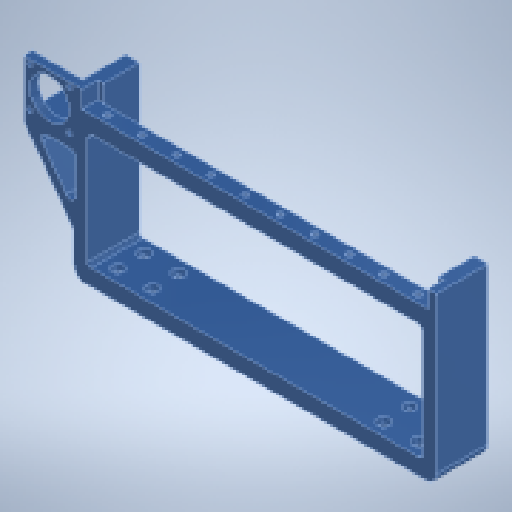
# Autodesk Inventor part: gantry_R
Saved by Autodesk Inventor 2024.1 (Build 281209000, 209)
## iProperties
Created: 2023-10-02
Part Number: gantry_R
Material: Generic
Document SubType Name: Modeling
Designer: l1534
Density: 1 g/cm^3
Appearance: Flaked Satin - Blue
Author: l1534
Autodesk Inventor part; units mm, degrees
ref_plane "YZ Plane" through (0, 0, 0) normal (1, 0, 0) x (0, 1, 0)
ref_plane "XZ Plane" through (0, 0, 0) normal (0, 1, 0) x (-1, 0, 0)
ref_plane "XY Plane" through (0, 0, 0) normal (0, 0, 1) x (1, 0, 0)
sketch "Sketch1" plane through (0, 0, 0) normal (0, 1, 0) x (-1, 0, 0)
  line L0 (96.4528, 98.5481) -> (-113.5472, 98.5481)
  line L1 (-113.5472, 98.5481) -> (-113.5472, 68.5481)
  line L2 (-113.5472, 68.5481) -> (96.4528, 68.5481)
  line L3 (96.4528, 68.5481) -> (96.4528, 98.5481)
  point P0 (0, 0)
  dimension "d0" = 210
  dimension "d1" = 30
  constraints: 8 end point, 2 parallel, 1 horizontal, 1 perpendicular
  measures "d0" distance of L1.end L2.end
  measures "d1" distance of L2.end L0.start
extrude "Extrusion1" add sketch "Sketch1" along normal blind 9.5
sketch "Sketch2" plane through (0, 9.5, 0) normal (0, 1, 0) x (1, 0, 0)
  line L0 (-96.4528, -68.5481) -> (-96.4528, -98.5481) projected
  line L1 (-96.4528, -98.5481) -> (-88.4528, -98.5481)
  line L2 (-88.4528, -98.5481) -> (-88.4528, -68.5481)
  line L3 (-88.4528, -68.5481) -> (-96.4528, -68.5481)
  line L4 (-96.4528, -68.5481) -> (-96.4528, -98.5481)
  line L5 (113.5472, -98.5481) -> (113.5472, -68.5481) projected
  line L6 (113.5472, -98.5481) -> (105.5472, -98.5481)
  line L7 (105.5472, -98.5481) -> (105.5472, -68.5481)
  line L8 (105.5472, -68.5481) -> (113.5472, -68.5481)
  line L9 (113.5472, -68.5481) -> (113.5472, -98.5481)
  point P0 (0, 0)
  point P1 (-96.4528, -68.5481)
  point P2 (-96.4528, -68.5481)
  dimension "d4" = 8
  dimension "d5" = 8
  dimension "d6" = 30
  constraints: 16 end point, 4 parallel, 2 horizontal, 2 perpendicular, 1 point on line
  measures "d4" distance of L2.end L3.end
  measures "d5" distance of L7.end L8.end
  measures "d6" distance between parallel lines of L6 L8
extrude "Extrusion2" add sketch "Sketch2" along normal blind 87
sketch "Sketch3" plane through (0, 9.5, 0) normal (0, 1, 0) x (1, 0, 0)
  circle A0 centre (95.5472, -91.0481) radius 1.55
  circle A1 centre (95.5472, -76.0481) radius 1.55
  circle A2 centre (-78.4528, -76.0481) radius 1.55
  circle A3 centre (-78.4528, -91.0481) radius 1.55
  circle A4 centre (75.5472, -91.0481) radius 1.55
  circle A5 centre (75.5472, -76.0481) radius 1.55
  circle A6 centre (-58.4528, -91.0481) radius 1.55
  circle A7 centre (-58.4528, -76.0481) radius 1.55
  line L0 (-88.4528, -98.5481) -> (105.5472, -98.5481) projected
  line L1 (105.5472, -68.5481) -> (105.5472, -98.5481) projected
  line L2 (-88.4528, -98.5481) -> (-88.4528, -68.5481) projected
  point P0 (0, 0)
  dimension "d9" = 3.1
  dimension "d10" = 3.1
  dimension "d11" = 3.1
  dimension "d12" = 3.1
  dimension "d13" = 3.1
  dimension "d14" = 3.1
  dimension "d15" = 3.1
  dimension "d16" = 3.1
  dimension "d17" = 20
  dimension "d18" = 15
  dimension "d19" = 20
  dimension "d20" = 15
  dimension "d21" = 7.5
  dimension "d22" = 7.5
  dimension "d23" = 10
  dimension "d24" = 10
  dimension "d25" = 7.5
  dimension "d26" = 7.5
  dimension "d27" = 10
  dimension "d28" = 10
  dimension "d29" = 15
  dimension "d30" = 20
  dimension "d31" = 15
  dimension "d32" = 20
  constraints: 8 centre point
  measures "d9" diameter of A0
  measures "d10" diameter of A1
  measures "d11" diameter of A3
  measures "d12" diameter of A2
  measures "d13" diameter of A7
  measures "d14" diameter of A6
  measures "d15" diameter of A4
  measures "d16" diameter of A5
  measures "d17" distance of A0.centre A4.centre
  measures "d18" distance of A5.centre A4.centre
  measures "d19" distance of A5.centre A1.centre
  measures "d20" distance of A1.centre A0.centre
  measures "d21" distance from line of L0 A0.centre
  measures "d22" distance from line of L0 A4.centre
  measures "d23" distance from line of L1 A0.centre
  measures "d24" distance from line of L1 A1.centre
  measures "d25" distance from line of L0 A3.centre
  measures "d26" distance from line of L0 A6.centre
  measures "d27" distance from line of L2 A3.centre
  measures "d28" distance from line of L2 A2.centre
  measures "d29" distance of A3.centre A2.centre
  measures "d30" distance of A3.centre A6.centre
  measures "d31" distance of A6.centre A7.centre
  measures "d32" distance of A2.centre A7.centre
extrude "Extrusion3" cut sketch "Sketch3" against normal through all
chamfer "Chamfer1" distance 2 angle 45 8 edges at (93.9972, 9.5, 91.0481) (93.9972, 9.5, 76.0481) (73.9972, 9.5, 76.0481) (73.9972, 9.5, 91.0481) (-60.0028, 9.5, 91.0481) (-80.0028, 9.5, 91.0481) (-80.0028, 9.5, 76.0481) (-60.0028, 9.5, 76.0481)
fillet "Fillet1" radius 2 2 edges at (105.5472, 9.5, 83.5481) (-88.4528, 9.5, 83.5481)
fillet "Fillet2" radius 6 2 edges at (113.5472, 0, 83.5481) (-96.4528, 0, 83.5481)
sketch "Sketch4" plane through (-86.4528, 9.5, 98.5481) normal (0, 0, 1) x (1, 0, 0)
  line L0 (-2, 2) -> (-2, 87) projected
  line L1 (192, 2) -> (192, 87) projected
  line L2 (-2, 77) -> (192, 77)
  line L3 (192, 77) -> (192, 67)
  line L4 (192, 67) -> (-2, 67)
  line L5 (-2, 67) -> (-2, 77)
  line L6 (-10, 87) -> (-2, 87) projected
  point P0 (86.4528, -9.5)
  point P1 (-2, 67)
  point P2 (192, 77)
  dimension "d40" = 10
  dimension "d41" = 10
  constraints: 8 end point, 2 parallel, 2 point on line, 1 horizontal, 1 perpendicular
  measures "d40" distance between parallel lines of L6 L2
  measures "d41" distance between parallel lines of L4 L2
extrude "Extrusion4" add sketch "Sketch4" against normal blind 9
sketch "Sketch5" plane through (0, 96.5, 0) normal (0, 1, 0) x (1, 0, 0)
  line L0 (105.5472, -98.5481) -> (105.5472, -68.5481) projected
  line L1 (105.5472, -98.5481) -> (108.7472, -98.5481)
  line L2 (108.7472, -98.5481) -> (108.7472, -89.3481)
  line L3 (108.7472, -89.3481) -> (105.5472, -89.3481)
  line L4 (105.5472, -89.3481) -> (105.5472, -98.5481)
  line L5 (-88.4528, -98.5481) -> (-88.4528, -68.5481) projected
  line L6 (-88.4528, -98.5481) -> (-91.6528, -98.5481)
  line L7 (-91.6528, -98.5481) -> (-91.6528, -89.3481)
  line L8 (-91.6528, -89.3481) -> (-88.4528, -89.3481)
  line L9 (-88.4528, -89.3481) -> (-88.4528, -98.5481)
  point P0 (0, 0)
  dimension "d44" = 3.2
  dimension "d45" = 9.2
  dimension "d46" = 3.2
  dimension "d47" = 9.2
  constraints: 16 end point, 4 parallel, 2 horizontal, 2 perpendicular
  measures "d44" distance of L5.start L6.end
  measures "d45" distance of L6.end L7.end
  measures "d46" distance of L0.start L1.end
  measures "d47" distance of L1.end L2.end
extrude "Extrusion5" cut sketch "Sketch5" against normal up to surface (10 mm away)
sketch "Sketch6" plane through (-88.4528, 86.5, 89.5481) normal (0, 1, 0) x (1, 0, 0)
  circle A0 centre (187, -4.5) radius 1.3
  line L0 (197.2, -9) -> (-3.2, -9) projected
  line L1 (197.2, 0.2) -> (197.2, -9) projected
  circle A1 centre (167, -4.5) radius 1.3
  circle A2 centre (147, -4.5) radius 1.3
  circle A3 centre (127, -4.5) radius 1.3
  circle A4 centre (107, -4.5) radius 1.3
  circle A5 centre (87, -4.5) radius 1.3
  circle A6 centre (67, -4.5) radius 1.3
  circle A7 centre (47, -4.5) radius 1.3
  circle A8 centre (27, -4.5) radius 1.3
  circle A9 centre (7, -4.5) radius 1.3
  point P0 (88.4528, 89.5481)
  dimension "d50" = 2.6
  dimension "d51" = 4.5
  dimension "d52" = 10.2
  dimension "d55" = 20
  constraints: 10 centre point, 1 horizontal, 18 other
  measures "d50" diameter of A0
  measures "d51" distance from line of L0 A0.centre
  measures "d52" distance from line of L1 A0.centre
  measures "d55" distance of A0.centre A1.centre
extrude "Extrusion6" cut sketch "Sketch6" against normal up to surface (10 mm away)
chamfer "Chamfer2" distance 0.5 angle 45 10 edges at (97.2472, 86.5, 94.0481) (77.2472, 86.5, 94.0481) (57.2472, 86.5, 94.0481) (37.2472, 86.5, 94.0481) (17.2472, 86.5, 94.0481) (-2.7528, 86.5, 94.0481) (-22.7528, 86.5, 94.0481) (-42.7528, 86.5, 94.0481) (-62.7528, 86.5, 94.0481) (-82.7528, 86.5, 94.0481)
sketch "Sketch7" plane through (-96.4528, 96.5, 68.5481) normal (-1, 0, 0) x (0, 0, 1)
  line L0 (0, 0) -> (30, 0) projected
  line L1 (30, 0) -> (25, 0)
  line L2 (25, 0) -> (25, -33)
  line L3 (25, -33) -> (30, -33)
  line L4 (30, -33) -> (30, 0)
  point P0 (-68.5481, -96.5)
  dimension "d65" = 5
  dimension "d66" = 33
  constraints: 8 end point, 2 parallel, 1 horizontal, 1 perpendicular
  measures "d65" distance of L2.end L3.end
  measures "d66" distance of L3.end L0.end
extrude "Extrusion7" add sketch "Sketch7" along normal blind 29
sketch "Sketch8" plane through (-96.4528, 6, 68.5481) normal (-1, 0, 0) x (0, 0, 1)
  line L0 (30, 57.5) -> (25, 57.5) projected
  line L1 (0, 5.5) -> (0, 90.5) projected
  line L2 (25, 57.5) -> (0, 57.5)
  line L3 (0, 57.5) -> (0, 62.3)
  line L4 (0, 62.3) -> (25, 62.3)
  line L5 (25, 62.3) -> (25, 57.5)
  point P0 (-68.5481, -6)
  point P1 (0, 57.5)
  dimension "d69" = 4.8
  constraints: 8 end point, 2 parallel, 1 horizontal, 1 perpendicular, 1 point on line
  measures "d69" distance between parallel lines of L2 L4
extrude "Extrusion8" add sketch "Sketch8" along normal blind 29
sketch "Sketch9" plane through (-96.4528, 96.5, 93.5481) normal (0, 0, -1) x (-1, 0, 0)
  circle A0 centre (14.1, -14.1) radius 11.5
  line L0 (0, -28.2) -> (29, -28.2) projected
  line L1 (0, -28.2) -> (0, 0) projected
  point P0 (-96.4528, -96.5)
  dimension "d40" = 10
  dimension "d72" = 23
  dimension "d73" = 14.1
  dimension "d74" = 14.1
  constraints: 1 centre point
  measures "d72" diameter of A0
  measures "d73" distance from line of L0 A0.centre
  measures "d74" distance from line of L1 A0.centre
extrude "Extrusion9" cut sketch "Sketch9" against normal through all
fillet "Fillet4" radius 3 2 edges at (105.5472, 76.5, 94.0481) (-88.4528, 76.5, 94.0481)
sketch "Sketch10" plane through (103.5472, 9.5, 68.5481) normal (0, 0, -1) x (-1, 0, 0)
  line L0 (200, 54) -> (229, 54) projected
  line L1 (200, 54) -> (229, 54)
  line L2 (229, 54) -> (200, 14)
  line L3 (200, -3.5) -> (200, 54) projected
  line L4 (200, 54) -> (200, 14)
  point P0 (103.5472, -9.5)
  dimension "d79" = 40
  constraints: 6 end point, 1 horizontal, 1 perpendicular, 1 point on line
  measures "d79" distance from line of L0 L2.end
extrude "Extrusion10" add sketch "Sketch10" against normal up to surface (30 mm away)
sketch "Sketch11" plane through (103.5472, 9.5, 68.5481) normal (0, 0, -1) x (-1, 0, 0)
  line L0 (222, 54) -> (199, 54)
  line L1 (199, 54) -> (199, 22.2759)
  line L2 (199, 22.2759) -> (222, 54)
  line L3 (200, 58.8) -> (229, 58.8) projected
  line L4 (192, 2) -> (192, 87) projected
  line L5 (200, 14) -> (229, 54) projected
  point P0 (103.5472, -9.5)
  dimension "d82" = 4.8
  dimension "d83" = 7
  dimension "d85" = 23
  constraints: 6 end point, 1 horizontal, 1 parallel, 1 perpendicular
  measures "d82" distance between parallel lines of L3 L0
  measures "d83" distance between parallel lines of L4 L1
  measures "d85" distance of L0.start L0.end
extrude "Extrusion11" cut sketch "Sketch11" against normal through all
fillet "Fillet5" radius 3 3 edges at (-95.4528, 63.5, 83.5481) (-95.4528, 31.7759, 83.5481) (-118.4528, 63.5, 83.5481)
fillet "Fillet6" radius 6 1 edges at (-96.4528, 23.5, 83.5481)
sketch "Sketch12" plane through (-90.4528, 0, 98.5481) normal (0, 0, 1) x (1, 0, 0)
  circle A0 centre (-31.6, 93.9) radius 1.3
  circle A1 centre (-8.6, 93.9) radius 1.3
  circle A2 centre (-8.6, 70.9) radius 1.3
  circle A3 centre (-31.6, 70.9) radius 1.3
  circle A4 centre (-20.1, 82.4) radius 11.5 projected
  point P0 (90.4528, 0)
  dimension "d90" = 2.6
  dimension "d91" = 2.6
  dimension "d92" = 2.6
  dimension "d93" = 2.6
  dimension "d94" = 11.5
  dimension "d95" = 11.5
  dimension "d96" = 11.5
  dimension "d97" = 11.5
  dimension "d98" = 11.5
  dimension "d99" = 11.5
  dimension "d100" = 11.5
  dimension "d101" = 11.5
  constraints: 4 centre point
  measures "d90" diameter of A0
  measures "d91" diameter of A1
  measures "d92" diameter of A3
  measures "d93" diameter of A2
  measures "d94" horizontal distance of A4.centre A0.centre
  measures "d95" horizontal distance of A4.centre A0.centre
  measures "d96" horizontal distance of A4.centre A1.centre
  measures "d97" horizontal distance of A4.centre A1.centre
  measures "d98" horizontal distance of A4.centre A3.centre
  measures "d99" horizontal distance of A4.centre A3.centre
  measures "d100" horizontal distance of A4.centre A2.centre
  measures "d101" horizontal distance of A4.centre A2.centre
extrude "Extrusion12" cut sketch "Sketch12" against normal through all contours A0 | A1 | A2 | A3
body "Solid1"
